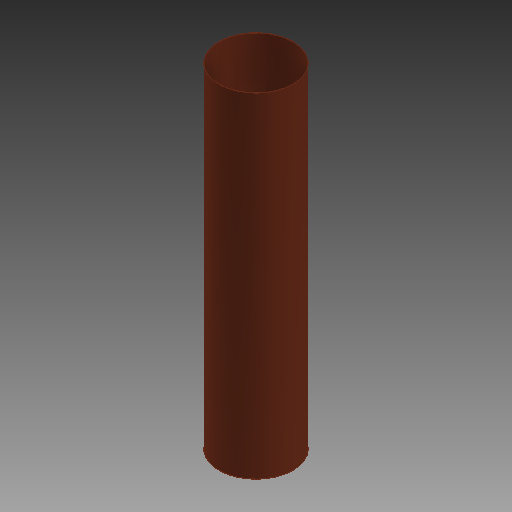
# Autodesk Inventor part: Coil
Saved by Autodesk Inventor 2019 (Build 230136000, 136)
## iProperties
Created: 2018-04-27
Part Number: Coil
Material: Copper
Document SubType Name: Modeling
Designer: Phil Erle
Density: 8.94 g/cm^3
Appearance: Copper - Satin
Author: Phil Erle
Autodesk Inventor part; units mm, degrees
ref_plane "YZ Plane" through (0, 0, 0) normal (1, 0, 0) x (0, 1, 0)
ref_plane "XZ Plane" through (0, 0, 0) normal (0, 1, 0) x (-1, 0, 0)
ref_plane "XY Plane" through (0, 0, 0) normal (0, 0, 1) x (1, 0, 0)
sketch "Sketch1" plane through (0, 0, 0) normal (0, 0, 1) x (1, 0, 0)
  circle A0 centre (0, 0) radius 55
  circle A1 centre (0, 0) radius 55.3
  dimension "d0" = 110
  dimension "d1" = 0.3
  constraints: 2 centre point, 2 coincident
  measures "d0" diameter of A0
  measures "d1" radial gap between concentric circles of A0 A1
extrude "Extrusion1" add sketch "Sketch1" along normal blind 500
body "Solid1"
